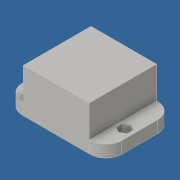
# Autodesk Inventor part: kaltgeraete
Saved by Autodesk Inventor 2016 (Build 200138000, 138)
## iProperties
Created: 2015-10-23
Part Number: kaltgeraete
Material: Generisch
Document SubType Name: Modeling
Designer: 4ndreas
Density: 1 g/cm^3
Appearance: Vorgabe
Author: 4ndreas
Autodesk Inventor part; units mm, degrees
ref_plane "YZ Plane" through (0, 0, 0) normal (1, 0, 0) x (0, 1, 0)
ref_plane "XZ Plane" through (0, 0, 0) normal (0, 1, 0) x (-1, 0, 0)
ref_plane "XY Plane" through (0, 0, 0) normal (0, 0, 1) x (1, 0, 0)
sketch "Skizze1" plane through (0, 0, 0) normal (0, 0, 1) x (1, 0, 0)
  line L0 (-25, -14) -> (25, -14)
  line L1 (25, -14) -> (25, 14)
  line L2 (25, 14) -> (-25, 14)
  line L3 (-25, 14) -> (-25, -14)
  line L4 (-25, -14) -> (25, 14) construction
  line L5 (25, -14) -> (-25, 14) construction
  line L6 (-13.5, -10) -> (13.5, -10)
  line L7 (13.5, -10) -> (13.5, 10)
  line L8 (13.5, 10) -> (-13.5, 10)
  line L9 (-13.5, 10) -> (-13.5, -10)
  line L10 (-13.5, -10) -> (13.5, 10) construction
  line L11 (13.5, -10) -> (-13.5, 10) construction
  circle A0 centre (-20.5, 0) radius 1.75
  circle A1 centre (20.5, 0) radius 1.75
  line L12 (-20.5, 0) -> (20.5, 0) construction
  point P0 (0, 0)
  point P1 (0, 0)
  point P2 (0, 0)
  point P3 (0, 0)
  dimension "d0" = 50
  dimension "d1" = 20
  dimension "d2" = 27
  dimension "d3" = 41
  dimension "d4" = 3.5
  dimension "d5" = 28
  constraints: 26 end point, 10 midpoint, 5 parallel, 2 centre point, 2 horizontal, 2 perpendicular, 1 equal radius
  measures "d0" distance between parallel lines of L1 L3
  measures "d1" distance between parallel lines of L6 L8
  measures "d2" distance between parallel lines of L7 L9
  measures "d3" distance of L12.start L12.end
  measures "d4" diameter of A1
  measures "d5" distance between parallel lines of L0 L2
extrude "Extrusion1" add sketch "Skizze1" along normal blind 6
sketch "Skizze2" plane through (0, 0, 6) normal (0, 0, 1) x (1, 0, 0)
  line L0 (-13.5, -10) -> (-13.5, 10) projected
  line L1 (-13.5, 10) -> (13.5, 10) projected
  line L2 (13.5, 10) -> (13.5, -10) projected
  line L3 (13.5, -10) -> (-13.5, -10) projected
  circle A0 centre (20.5, 0) radius 1.75 projected
  circle A1 centre (-20.5, 0) radius 1.75 projected
  line L4 (-25, -14) -> (25, -14) projected
  line L5 (25, -14) -> (25, 14) projected
  line L6 (25, 14) -> (-25, 14) projected
  line L7 (-25, 14) -> (-25, -14) projected
  line L8 (-20.5, 3.1754) -> (-17.75, 1.5877)
  line L9 (-17.75, 1.5877) -> (-17.75, -1.5877)
  line L10 (-17.75, -1.5877) -> (-20.5, -3.1754)
  line L11 (-20.5, -3.1754) -> (-23.25, -1.5877)
  line L12 (-23.25, -1.5877) -> (-23.25, 1.5877)
  line L13 (-23.25, 1.5877) -> (-20.5, 3.1754)
  line L14 (20.5, 3.1754) -> (23.25, 1.5877)
  line L15 (23.25, 1.5877) -> (23.25, -1.5877)
  line L16 (23.25, -1.5877) -> (20.5, -3.1754)
  line L17 (20.5, -3.1754) -> (17.75, -1.5877)
  line L18 (17.75, -1.5877) -> (17.75, 1.5877)
  line L19 (17.75, 1.5877) -> (20.5, 3.1754)
  line L20 (-25, 14) -> (-25, -14) projected
  line L21 (25, -14) -> (25, 14) projected
  point P0 (0, 0)
  dimension "d8" = 5.5
  constraints: 24 end point, 3 parallel, 2 coincident, 26 other
  measures "d8" distance between parallel lines of L12 L9
extrude "Extrusion2" cut sketch "Skizze2" against normal blind 3 contours A0 | A1 | L8 L9 L10 L11 L12 L13 | L14 L15 L16 L17 L18 L19
sketch "Skizze3" plane through (0, 0, 6) normal (0, 0, 1) x (1, 0, 0)
  line L0 (-23.25, 1.5877) -> (-20.5, 3.1754) projected
  line L1 (-20.5, 3.1754) -> (-17.75, 1.5877) projected
  line L2 (-17.75, 1.5877) -> (-17.75, -1.5877) projected
  line L3 (-17.75, -1.5877) -> (-20.5, -3.1754) projected
  line L4 (-20.5, -3.1754) -> (-23.25, -1.5877) projected
  line L5 (-23.25, -1.5877) -> (-23.25, 1.5877) projected
  line L6 (17.75, 1.5877) -> (20.5, 3.1754) projected
  line L7 (20.5, 3.1754) -> (23.25, 1.5877) projected
  line L8 (23.25, 1.5877) -> (23.25, -1.5877) projected
  line L9 (23.25, -1.5877) -> (20.5, -3.1754) projected
  line L10 (20.5, -3.1754) -> (17.75, -1.5877) projected
  line L11 (17.75, -1.5877) -> (17.75, 1.5877) projected
  line L12 (-13.5, -10) -> (-13.5, 10) projected
  line L13 (-13.5, 10) -> (13.5, 10) projected
  line L14 (13.5, 10) -> (13.5, -10) projected
  line L15 (13.5, -10) -> (-13.5, -10) projected
  line L16 (-25, -14) -> (25, -14) projected
  line L17 (25, -14) -> (25, 14) projected
  line L18 (25, 14) -> (-25, 14) projected
  line L19 (-25, 14) -> (-25, -14) projected
  line L20 (-16.5, -14) -> (16.5, -14)
  line L21 (16.5, -14) -> (16.5, 14)
  line L22 (16.5, 14) -> (-16.5, 14)
  line L23 (-16.5, 14) -> (-16.5, -14)
  line L24 (-16.5, -14) -> (16.5, 14) construction
  line L25 (16.5, -14) -> (-16.5, 14) construction
  point P0 (0, 0)
  dimension "d11" = 3
  constraints: 12 end point, 2 midpoint, 2 parallel, 1 horizontal, 1 perpendicular, 1 point on line
  measures "d11" distance between parallel lines of L23 L12
extrude "Extrusion3" add sketch "Skizze3" along normal blind 14 contours L23 L18 L21 L16
sketch "Skizze4" plane through (0, 0, 20) normal (0, 0, 1) x (1, 0, 0)
  line L0 (-13.5, 10) -> (13.5, 10) projected
  line L1 (13.5, 10) -> (13.5, -10) projected
  line L2 (13.5, -10) -> (-13.5, -10) projected
  line L3 (-13.5, -10) -> (-13.5, 10) projected
  line L4 (16.5, 14) -> (-16.5, 14) projected
  line L5 (-16.5, 14) -> (-16.5, -14) projected
  line L6 (-16.5, -14) -> (16.5, -14) projected
  line L7 (16.5, -14) -> (16.5, 14) projected
  point P0 (0, 0)
extrude "Extrusion4" add sketch "Skizze4" along normal blind 2 contours L0 L1 L2 L3 | L7 L6 L5 L4
sketch "Skizze5" plane through (-13.5, 10, 0) normal (0, -1, 0) x (1, 0, 0)
  line L0 (27, 0) -> (0, 0) projected
  line L1 (27, 0) -> (27, 20) projected
  line L2 (0, 20) -> (27, 20) projected
  line L3 (0, 0) -> (0, 20) projected
  line L4 (38.5, 0) -> (-11.5, 0) projected
  line L5 (-11.5, 0) -> (-11.5, 6) projected
  line L6 (-3, 6) -> (-11.5, 6) projected
  line L7 (-3, 6) -> (-3, 22) projected
  line L8 (30, 22) -> (-3, 22) projected
  line L9 (30, 6) -> (30, 22) projected
  line L10 (38.5, 6) -> (30, 6) projected
  line L11 (38.5, 0) -> (38.5, 6) projected
  line L12 (0, 6) -> (27, 6)
  line L13 (27, 6) -> (27, 20)
  line L14 (27, 20) -> (0, 20)
  line L15 (0, 20) -> (0, 6)
  line L16 (0, 6) -> (27, 20) construction
  line L17 (27, 6) -> (0, 20) construction
  point P0 (13.5, 0)
  point P1 (13.5, 13)
  constraints: 12 end point, 2 collinear, 2 midpoint, 2 parallel, 1 horizontal, 1 perpendicular
extrude "Extrusion5" cut sketch "Skizze5" against normal through all contours L12 L3 L2 L1
sketch "Skizze7" plane through (-25, 14, 0) normal (0, 1, 0) x (1, 0, 0)
  line L0 (38.5, 0) -> (38.5, -6) projected
  line L1 (11.5, -20) -> (11.5, -6) projected
  line L2 (11.5, -6) -> (38.5, -6) projected
  line L3 (38.5, -6) -> (38.5, -20) projected
  line L4 (38.5, -20) -> (11.5, -20) projected
  line L5 (50, 0) -> (0, 0) projected
  line L6 (0, 0) -> (0, -6) projected
  line L7 (8.5, -6) -> (0, -6) projected
  line L8 (8.5, -6) -> (8.5, -22) projected
  line L9 (41.5, -22) -> (8.5, -22) projected
  line L10 (41.5, -6) -> (41.5, -22) projected
  line L11 (50, -6) -> (41.5, -6) projected
  line L12 (50, 0) -> (50, -6) projected
  point P0 (25, 0)
extrude "Extrusion6" add sketch "Skizze7" along normal blind 6
chamfer "Fase1" distance 5 angle 45 1 edges at (0, 10, 6)
fillet "Rundung1" radius 8 4 edges at (25, -14, 3) (25, 20, 3) (-25, -14, 3) (-25, 20, 3)
